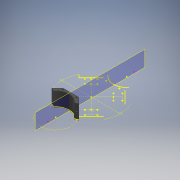
# Autodesk Inventor part: catch_v2
Saved by Autodesk Inventor 2020 (Build 240168000, 168)
## iProperties
Created: 2024-11-02
Part Number: catch_v2
Material: Полиэтилен, низкая плотность
Document SubType Name: Modeling
Designer: Ivan
Density: 0.894 g/cm^3
Appearance: Типовые
Mass: 48.1181 g
Surface Area: 138.225 cm^2
Volume: 53.8234 cm^3
Author: Ivan
Autodesk Inventor part; units mm, degrees
ref_plane "YZ Plane" through (0, 0, 0) normal (1, 0, 0) x (0, 1, 0)
ref_plane "XZ Plane" through (0, 0, 0) normal (0, 1, 0) x (-1, 0, 0)
ref_plane "XY Plane" through (0, 0, 0) normal (0, 0, 1) x (1, 0, 0)
derived "floor_v2.ipt"
sketch "Эскиз2" plane through (0, 0, 0) normal (0, 1, 0) x (1, 0, 0)
  circle A0 centre (0, 0) radius 107.5
  circle A1 centre (0, 0) radius 104
  line L0 (0, 0) -> (104, 0) construction
  line L1 (0, 0) -> (0, -104) construction
  line L2 (0, 0) -> (-104, 0) construction
  line L3 (0, 0) -> (0, 104) construction
  line L4 (104, 0) -> (0, -104) construction
  line L5 (0, 104) -> (-104, 0) construction
  line L6 (0, -104) -> (-104, 0) construction
  line L7 (104, 0) -> (0, 104) construction
  line L8 (0, 0) -> (-73.5391, -73.5391) construction
  line L9 (0, 0) -> (73.5391, -73.5391) construction
  line L10 (0, 0) -> (73.5391, 73.5391) construction
  line L11 (0, 0) -> (-73.5391, 73.5391) construction
  line L12 (-38.4471, -82.2877) -> (-82.2877, -38.4471)
  line L13 (-38.4471, -82.2877) -> (-48.2758, -92.1165)
  line L14 (-82.2877, -38.4471) -> (-92.1165, -48.2758)
  line L15 (92.1165, -48.2758) -> (82.2877, -38.4471)
  line L16 (82.2877, -38.4471) -> (38.4471, -82.2877)
  line L17 (38.4471, -82.2877) -> (48.2758, -92.1165)
  line L18 (48.2758, 92.1165) -> (38.4471, 82.2877)
  line L19 (38.4471, 82.2877) -> (82.2877, 38.4471)
  line L20 (82.2877, 38.4471) -> (92.1165, 48.2758)
  line L21 (-48.2758, 92.1165) -> (-38.4471, 82.2877)
  line L22 (-38.4471, 82.2877) -> (-82.2877, 38.4471)
  line L23 (-82.2877, 38.4471) -> (-92.1165, 48.2758)
  line L24 (0, -107.5) -> (0, -79.5) construction
  circle A2 centre (0, -116.5) radius 37 construction
  circle A3 centre (0, -127) radius 47.5
  line L25 (0, 107.5) -> (0, 79.5) construction
  circle A4 centre (0, 127) radius 47.5
  line L26 (-92.1165, 48.2758) -> (-94.7051, 50.8645)
  line L27 (-48.2758, 92.1165) -> (-50.8645, 94.7051)
  line L28 (48.2758, 92.1165) -> (50.8645, 94.7051)
  line L29 (92.1165, 48.2758) -> (94.7051, 50.8645)
  line L30 (92.1165, -48.2758) -> (94.7051, -50.8645)
  line L31 (48.2758, -92.1165) -> (50.8645, -94.7051)
  line L32 (-92.1165, -48.2758) -> (-94.7051, -50.8645)
  line L33 (-48.2758, -92.1165) -> (-50.8645, -94.7051)
  point P0 (-52, -52)
  point P1 (-52, 52)
  point P2 (52, 52)
  point P3 (52, -52)
  point P4 (-60.3674, -60.3674)
  point P5 (60.3674, -60.3674)
  point P6 (60.3674, 60.3674)
  point P7 (-60.3674, 60.3674)
  point P8 (-36.9892, -97.1998)
  point P9 (36.9892, -97.1998)
  point P10 (36.9892, 97.1998)
  point P11 (-36.9892, 97.1998)
sketch "Эскиз3" plane through (0, 2, 0) normal (0, -1, 0) x (-1, 0, 0)
  line L0 (33.8509, 77.6915) -> (77.6915, 33.8509) construction
  line L1 (55.7712, 55.7712) -> (0, 0) construction
  line L2 (44.4575, 67.0849) -> (67.0849, 44.4575) construction
  circle A0 centre (44.4575, 67.0849) radius 1.5
  circle A1 centre (67.0849, 44.4575) radius 1.5
  line L3 (28.3991, 51.0265) -> (51.0265, 28.3991) construction
  circle A2 centre (28.3991, 51.0265) radius 1.5
  circle A3 centre (51.0265, 28.3991) radius 1.5
  line L4 (44.4575, -67.0849) -> (67.0849, -44.4575) construction
  line L5 (28.3991, -51.0265) -> (51.0265, -28.3991) construction
  line L6 (55.7712, -55.7712) -> (0, 0) construction
  line L7 (-55.7712, -55.7712) -> (0, 0) construction
  line L8 (-28.3991, -51.0265) -> (-51.0265, -28.3991) construction
  line L9 (-44.4575, -67.0849) -> (-67.0849, -44.4575) construction
  line L10 (-55.7712, 55.7712) -> (0, 0) construction
  line L11 (-51.0265, 28.3991) -> (-28.3991, 51.0265) construction
  line L12 (-67.0849, 44.4575) -> (-44.4575, 67.0849) construction
  circle A4 centre (-44.4575, 67.0849) radius 1.5
  circle A5 centre (-67.0849, 44.4575) radius 1.5
  circle A6 centre (-28.3991, 51.0265) radius 1.5
  circle A7 centre (-51.0265, 28.3991) radius 1.5
  circle A8 centre (-44.4575, -67.0849) radius 1.5
  circle A9 centre (-67.0849, -44.4575) radius 1.5
  circle A10 centre (-51.0265, -28.3991) radius 1.5
  circle A11 centre (-28.3991, -51.0265) radius 1.5
  circle A12 centre (44.4575, -67.0849) radius 1.5
  circle A13 centre (28.3991, -51.0265) radius 1.5
  circle A14 centre (51.0265, -28.3991) radius 1.5
  circle A15 centre (67.0849, -44.4575) radius 1.5
  line L13 (-38.4471, -82.2877) -> (-82.2877, -38.4471)
  line L14 (82.2877, -38.4471) -> (38.4471, -82.2877)
  line L15 (38.4471, 82.2877) -> (82.2877, 38.4471)
  line L16 (-82.2877, 38.4471) -> (-38.4471, 82.2877)
  line L17 (82.2877, 38.4471) -> (92.1165, 48.2758)
  point P0 (39.7128, 39.7128)
  point P1 (-39.7128, -39.7128)
  point P2 (39.7128, -39.7128)
  point P3 (-39.7128, 39.7128)
  point P4 (-40.1306, -40.1306)
sketch "Эскиз6" plane through (0, 2, 0) normal (0, -1, 0) x (-1, 0, 0)
  arc A0 (36.9892, -97.1998) -> (-36.9892, -97.1998) centre (0, -127) ccw
  arc A1 (-36.9892, 97.1998) -> (36.9892, 97.1998) centre (0, 127) ccw
  point P0 (-0.0301, 154.5629)
  point P1 (-0.0412, -154.5628)
sketch "Эскиз8" plane through (0, 2, 0) normal (0, 1, 0) x (1, 0, 0)
  arc A0 (-48.2758, -92.1165) -> (-36.9892, -97.1998) centre (0, 0) ccw
  arc A1 (36.9892, -97.1998) -> (48.2758, -92.1165) centre (0, 0) ccw
  arc A2 (36.9892, -97.1998) -> (-36.9892, -97.1998) centre (0, -127) ccw
  circle A3 centre (0, -127) radius 55.4164 construction
  circle A4 centre (-23.8556, -76.9811) radius 1.5
  circle A5 centre (23.8556, -76.9811) radius 1.5
  circle A6 centre (-28.3991, -51.0265) radius 1.5 construction
  circle A7 centre (-51.0265, -28.3991) radius 1.5 construction
  circle A8 centre (-67.0849, -44.4575) radius 1.5 construction
  circle A9 centre (-44.4575, -67.0849) radius 1.5 construction
  circle A10 centre (-51.0265, -28.3991) radius 1.5 construction
  line L0 (-51.0265, -28.3991) -> (-28.3991, -51.0265) construction
  line L1 (-67.0849, -44.4575) -> (-44.4575, -67.0849) construction
  line L2 (-55.7712, -55.7712) -> (-39.7128, -39.7128) construction
  line L3 (-50.4184, -50.4184) -> (-23.8556, -76.9811) construction
  circle A11 centre (67.0849, -44.4575) radius 1.5 construction
  circle A12 centre (44.4575, -67.0849) radius 1.5 construction
  line L4 (44.4575, -67.0849) -> (67.0849, -44.4575) construction
  arc A13 (-92.1165, 48.2758) -> (-92.1165, -48.2758) centre (0, 0) ccw construction
  line L5 (-104, 0) -> (104, 0) construction
  arc A14 (92.1165, -48.2758) -> (92.1165, 48.2758) centre (0, 0) ccw construction
  circle A15 centre (-23.8556, 76.9811) radius 1.5
  circle A16 centre (23.8556, 76.9811) radius 1.5
  point P0 (-44.5136, -93.9922)
  point P1 (-104, 0)
sketch "Эскиз5" plane through (0, 0, 0) normal (0, 1, 0) x (-1, 0, 0)
  arc A0 (-36.9892, 97.1998) -> (36.9892, 97.1998) centre (0, 127) ccw projected
  circle A1 centre (0, 0) radius 104 projected
  line L0 (38.4471, 82.2877) -> (48.2758, 92.1165) projected
  line L1 (-38.4471, 82.2877) -> (-48.2758, 92.1165) projected
  line L2 (38.4471, 82.2877) -> (28.1405, 71.9811)
  line L3 (-38.4471, 82.2877) -> (-28.1405, 71.9811)
  line L4 (28.1405, 71.9811) -> (-28.1405, 71.9811)
  line L5 (82.2877, 38.4471) -> (38.4471, 82.2877) projected
  circle A2 centre (23.8556, 76.9811) radius 1.5 projected
  circle A3 centre (-23.8556, 76.9811) radius 1.5 projected
  circle A4 centre (23.8556, 76.9811) radius 5 construction
  circle A5 centre (-23.8556, 76.9811) radius 5 construction
  dimension "d2" = 10
  dimension "d3" = 10
  constraints: 6 end point, 2 centre point, 2 coincident, 2 collinear, 1 horizontal, 1 perpendicular, 1 tangent
  measures "d2" diameter of A4
  measures "d3" diameter of A5
extrude "Выдавливание1" add sketch "Эскиз5" along normal blind 51.15 contours A0 A1 L0 L2 L4 L3 L1 | A2 | A3
sketch "Эскиз9" plane through (0, 51.15, 0) normal (0, 1, 0) x (1, 0, 0)
  circle A0 centre (-23.8556, -76.9811) radius 1.5 projected
  circle A1 centre (23.8556, -76.9811) radius 1.5 projected
  point P0 (0, 0)
hole "Отверстие1" at (-23.8556, 51.15, 76.9811) at (23.8556, 51.15, 76.9811) direction (0, -1, 0) diameter 4 depth 7
hole "Отверстие2" at (-23.8556, 0, 76.9811) at (23.8556, 0, 76.9811) direction (0, 1, 0) diameter 4 depth 7
fillet "Сопряжение1" radius 10 2 edges at (-28.1405, 25.575, 71.9811) (28.1405, 25.575, 71.9811)
ref_plane "РабПлоскость1" through (-36.9892, 0, 97.1998) normal (0.6637718, 0, -0.7479351) x (-0.7479351, 0, -0.6637718)
sketch "Эскиз10" plane through (-36.9892, 0, 97.1998) normal (0.6637718, 0, -0.7479351) x (-0.7479351, 0, -0.6637718)
  line L0 (0, 0) -> (0, 51.15) projected
  line L1 (0, 25.575) -> (21.6029, 25.575)
  circle A0 centre (6.19, 26) radius 2
  point P0 (36.853, 0)
  dimension "d21" = 4
  dimension "d22" = 6.19
  constraints: 2 end point, 1 centre point, 1 midpoint, 1 perpendicular
  measures "d21" diameter of A0
  measures "d22" distance from line of L0 A0.centre
extrude "Выдавливание2" cut sketch "Эскиз10" along normal blind 5 and the other way blind 5
ref_plane "РабПлоскость2" through (0, 0, 43.8406) normal (-1, 0, 0) x (0, 1, 0)
mirror "Зеркальное отражение1" about plane through (0, 0, 43.8406) normal (-1, 0, 0) of "Выдавливание2"
equation "\"d3\" = d2"
